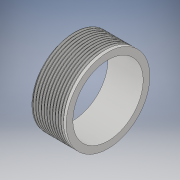
# Autodesk Inventor part: Thread_Imperial
Saved by Autodesk Inventor 2019 (Build 230136000, 136)
## iProperties
Created: 2019-04-30
Part Number: Thread_Imperial
Material: Generic
Document SubType Name: Modeling
Designer: rhabluet
Density: 1 g/cm^3
Appearance: Default
Author: rhabluet
Autodesk Inventor part; units mm, degrees
ref_plane "YZ Plane" through (0, 0, 0) normal (1, 0, 0) x (0, 1, 0)
ref_plane "XZ Plane" through (0, 0, 0) normal (0, 1, 0) x (-1, 0, 0)
ref_plane "XY Plane" through (0, 0, 0) normal (0, 0, 1) x (1, 0, 0)
sketch "Sketch2" plane through (0, 0, 0) normal (1, 0, 0) x (0, 1, 0)
  circle A0 centre (0, 0) radius 11.9062
  circle A1 centre (0, 0) radius 10
  dimension "d0" = 23.8125
  dimension "d3" = 20
  constraints: 2 centre point, 2 coincident
  measures "d0" diameter of A0
  measures "d3" diameter of A1
extrude "Extrusion2" add sketch "Sketch2" along normal blind 10
sketch "Sketch3" plane through (0, 0, 0) normal (0, 0, 1) x (1, 0, 0)
  line L0 (0, -16.6688) -> (0, 16.6688) construction
  line L1 (-0.3969, 11.9922) -> (-1.1906, 11.9922) construction
  line L2 (-1.1906, 11.9922) -> (-1.141, 11.9062) construction
  line L3 (-1.141, 11.9062) -> (-0.893, 11.4766)
  line L4 (-0.893, 11.4766) -> (-0.7937, 11.3048) construction
  line L5 (-0.7937, 11.3048) -> (-0.6945, 11.4766) construction
  line L6 (-0.6945, 11.4766) -> (-0.4465, 11.9062)
  line L7 (-0.4465, 11.9062) -> (-0.3969, 11.9922) construction
  line L8 (-1.141, 11.9062) -> (-0.4465, 11.9062)
  line L9 (-0.893, 11.4766) -> (-0.6945, 11.4766) construction
  arc A0 (-0.893, 11.4766) -> (-0.6945, 11.4766) centre (-0.7937, 11.5339) ccw
  line L10 (0, 11.9062) -> (0, -11.9062) projected
  point P0 (0, 0)
  point P1 (-0.7937, 11.9062)
  dimension "d6" = 60
  dimension "d7" = 0.7937
  dimension "d8" = 0.6945
  dimension "d9" = 0.1984
  dimension "d10" = 60
  dimension "d11" = 0.7937
  constraints: 18 end point, 6 point on line, 3 horizontal, 2 point on circle, 2 tangent, 1 centre point, 1 midpoint
  measures "d6" angle of L5 L4
  measures "d7" distance of L1.start L1.end
  measures "d8" distance of L2.end L6.end
  measures "d9" distance of L3.end L5.end
  measures "d10" angle of L8 L3
  measures "d11" distance of L10.start point (-0.794, 11.906)
coil "Coil1" sketch "Sketch3" operation cut axis through (-10, 0, 0) along (1, 0, 0) pitch 0.7937 turns 12.598425 hand right
equation "\"d7\" = pitch"
equation "\"d8\" = 0.875 * pitch"
equation "\"d9\" = 0.25 * pitch"
equation "\"d11\" = pitch"
equation "\"d12\" = pitch"
equation "\"pitch\" = 0.79375"
body "Solid2"
